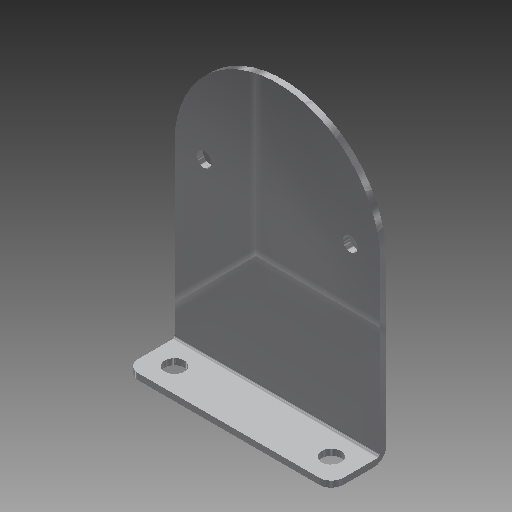
# Autodesk Inventor part: Pneumatics_VIAIR_00090_02
Saved by Autodesk Inventor 2017 (Build 210142000, 142)
## iProperties
Created: 2011-12-01
Part Number: Pneumatics_VIAIR_00090_02
Material: Generic
Document SubType Name: Modeling
Designer: Phillip
Density: 1 g/cm^3
Appearance: Aluminum - Polished
Author: Phillip
Autodesk Inventor part; units mm, degrees
ref_plane "YZ Plane" through (0, 0, 0) normal (1, 0, 0) x (0, 1, 0)
ref_plane "XZ Plane" through (0, 0, 0) normal (0, 1, 0) x (-1, 0, 0)
ref_plane "XY Plane" through (0, 0, 0) normal (0, 0, 1) x (1, 0, 0)
sketch "Sketch1" plane through (0, 0, 0) normal (0, 0, 1) x (1, 0, 0)
  circle A0 centre (0, 0) radius 26.797 projected
  line L0 (-26.797, -45.7454) -> (26.797, -45.7454)
  line L1 (-26.797, 0) -> (-26.797, -45.7454)
  line L2 (26.797, 0) -> (26.797, -45.7454)
  line L3 (-26.797, -45.7454) -> (26.797, -45.7454) projected
  point P0 (0, 0)
  constraints: 6 end point, 2 perpendicular, 2 point on circle, 2 tangent, 1 collinear
extrude "Extrusion1" add sketch "Sketch1" along normal blind 1.5875
sketch "Sketch2" plane through (0, 0, 1.5875) normal (0, 0, 1) x (1, 0, 0)
  line L0 (26.797, 0) -> (26.797, -45.7454) projected
  line L1 (-26.797, -45.7454) -> (26.797, -45.7454)
  line L2 (26.797, -45.7454) -> (26.797, -44.1579)
  line L3 (26.797, -44.1579) -> (-26.797, -44.1579)
  line L4 (-26.797, -44.1579) -> (-26.797, -45.7454)
  dimension "d2" = 1.5875
  constraints: 8 end point, 2 parallel, 1 horizontal, 1 perpendicular, 1 point on line
  measures "d2" distance between parallel lines of L1 L3
extrude "Extrusion2" add sketch "Sketch2" along normal blind 12.7
fillet "Fillet1" radius 3.175 2 edges at (-26.797, -44.9517, 14.2875) (26.797, -44.9517, 14.2875)
hole "Hole1" at (-20.447, -44.1579, 7.9375) direction (0, -1, 0) diameter 5.1054 end through all clearance for "Flat Head Machine Screw (82)" size "#10" standard "Ansi Unified Screw Threads"
fillet "Fillet2" radius 0.7937 1 edges at (0, -44.1579, 1.5875)
hole "Hole2" at (20.447, -44.1579, 7.9375) direction (0, -1, 0) diameter 5.1054 end through all clearance for "Flat Head Machine Screw (82)" size "#10" standard "Ansi Unified Screw Threads"
sketch "Sketch3" plane through (0, 0, 1.5875) normal (0, 0, 1) x (1, 0, 0)
  arc A0 (26.797, 0) -> (-26.797, 0) centre (0, 0) ccw projected
  point P0 (-19.05, 0)
  point P1 (19.05, 0)
  dimension "d26" = 19.05
  dimension "d27" = 19.05
  constraints: 2 horizontal alignment
  measures "d26" distance of point (-19.05, 0) A0.centre
  measures "d27" distance of point (19.05, 0) A0.centre
hole "Hole3" at (-19.05, 0, 1.5875) at (19.05, 0, 1.5875) direction (0, 0, -1) diameter 3.81 end through all clearance for "Flat Head Machine Screw (82)" size "#6" standard "Ansi Unified Screw Threads"
fillet "Fillet3" radius 3.175 1 edges at (0, -45.7454, 0)
equation "\"d27\" = d26"
body "Solid1"
